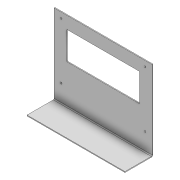
# Autodesk Inventor part: Display_Mount_A
Saved by Autodesk Inventor 2020 (Build 240168000, 168)
## iProperties
Created: 2021-12-05
Part Number: Display_Mount_A
Material: 一般
Document SubType Name: Sheet Metal
Designer: ken113
Density: 1 g/cm^3
Sheet Metal Rule: Default_mm
Appearance: 既定
Author: ken113
Autodesk Inventor part; units mm, degrees
ref_plane "YZ Plane" through (0, 0, 0) normal (1, 0, 0) x (0, 1, 0)
ref_plane "XZ Plane" through (0, 0, 0) normal (0, 1, 0) x (-1, 0, 0)
ref_plane "XY Plane" through (0, 0, 0) normal (0, 0, 1) x (1, 0, 0)
sketch "スケッチ1" plane through (0, 0, 0) normal (0, 0, 1) x (1, 0, 0)
  line L0 (175, -140) -> (-175, -140)
  line L1 (-175, -140) -> (-175, 140)
  line L2 (-175, 140) -> (175, 140)
  line L3 (175, 140) -> (175, -140)
  line L4 (175, -140) -> (-175, 140) construction
  line L5 (-175, -140) -> (175, 140) construction
  point P0 (0, 0)
  dimension "d0" = 280
  dimension "d1" = 350
  measures "d0" distance of L0.end L1.end
  measures "d1" distance of L1.end L2.end
extrude "プレート1" add sketch "スケッチ1" along normal blind 3
sketch "スケッチ2" plane through (175, -143, 6) normal (0, -1, 0) x (1, 0, 0)
  line L0 (-350, 0) -> (0, 0)
  line L1 (0, 0) -> (0, 94)
  line L2 (0, 94) -> (-350, 94)
  line L3 (-350, 94) -> (-350, 0)
  constraints: 6 end point, 1 horizontal, 1 perpendicular, 1 vertical
edge flange "フランジ1" height 100 angle 90 thickness 3 bend radius 3 thickness toward (0, -1, 0) relief straight relief width 3 relief depth 1.5 edges at (0, -140, 3) wall of the first edge with corners at (-175, -143, 6) (175, -143, 6) (175, -143, 100) (-175, -143, 100)
bend "曲げ1"
corner "コーナー1"
sketch "スケッチ3" plane through (0, 0, 3) normal (0, 0, 1) x (1, 0, 0)
  line L0 (150, -80) -> (-150, -80)
  line L1 (-150, -80) -> (-150, 120)
  line L2 (-150, 120) -> (150, 120)
  line L3 (150, 120) -> (150, -80)
  line L4 (150, -80) -> (-150, 120) construction
  line L5 (-150, -80) -> (150, 120) construction
  line L6 (175, -140) -> (-175, -140) projected
  point P0 (0, 0)
  point P1 (0, 20)
  dimension "d13" = 300
  dimension "d14" = 200
  dimension "d15" = 60
  constraints: 12 end point, 2 midpoint, 2 parallel, 1 horizontal, 1 perpendicular
  measures "d13" distance of L0.start L0.end
  measures "d14" distance of L0.end L1.end
  measures "d15" distance between parallel lines of L0 L6
hole "穴1" at (-150, 120, 3) at (-150, -80, 3) at (150, -80, 3) at (150, 120, 3) direction (0, 0, -1) diameter 6.2 depth 3 tip angle 118
sketch "スケッチ4" plane through (0, 0, 3) normal (0, 0, 1) x (1, 0, 0)
  line L0 (130, -3.8) -> (-130, -3.8)
  line L1 (-130, -3.8) -> (-130, 96.2)
  line L2 (-130, 96.2) -> (130, 96.2)
  line L3 (130, 96.2) -> (130, -3.8)
  line L4 (130, -3.8) -> (-130, 96.2) construction
  line L5 (-130, -3.8) -> (130, 96.2) construction
  circle A0 centre (-150, 120) radius 3.1 projected
  point P0 (0, 0)
  point P1 (0, 46.2)
  point P2 (0, 46.2)
  dimension "d23" = 100
  dimension "d24" = 23.8
  dimension "d25" = 260
  constraints: 12 end point, 3 midpoint, 2 parallel, 1 horizontal, 1 perpendicular, 1 vertical alignment
  measures "d23" distance of L2.end L0.start
  measures "d24" distance from line of L2 A0.centre
  measures "d25" distance of L1.end L2.end
extrude "押し出し1" cut sketch "スケッチ4" against normal through all contours L0 L1 L2 L3
fillet "フィレット1" radius 2 4 edges at (130, -3.8, 1.5) (130, 96.2, 1.5) (-130, 96.2, 1.5) (-130, -3.8, 1.5)
equation "\"d21\" = Thickness"
equation "\"d2\" = Thickness"
equation "\"d3\" = BendReliefWidth"
equation "\"d4\" = BendReliefDepth"
equation "\"d5\" = MinimumRemnant"
equation "\"d6\" = TransitionRadius"
equation "\"d9\" = BendRadius"
equation "\"d10\" = CornerReliefSize"
equation "\"d11\" = GapSize"
equation "\"d12\" = JacobiRadiusSize"
equation "\"BendRadius\" = Thickness"
equation "\"BendReliefWidth\" = Thickness"
equation "\"BendReliefDepth\" = 0.5 * Thickness"
equation "\"CornerReliefSize\" = 4 * Thickness"
equation "\"MinimumRemnant\" = 2 * Thickness"
equation "\"TransitionRadius\" = BendRadius"
equation "\"JacobiRadiusSize\" = BendRadius"
equation "\"GapSize\" = Thickness"
equation "\"Thickness\" = 3"
